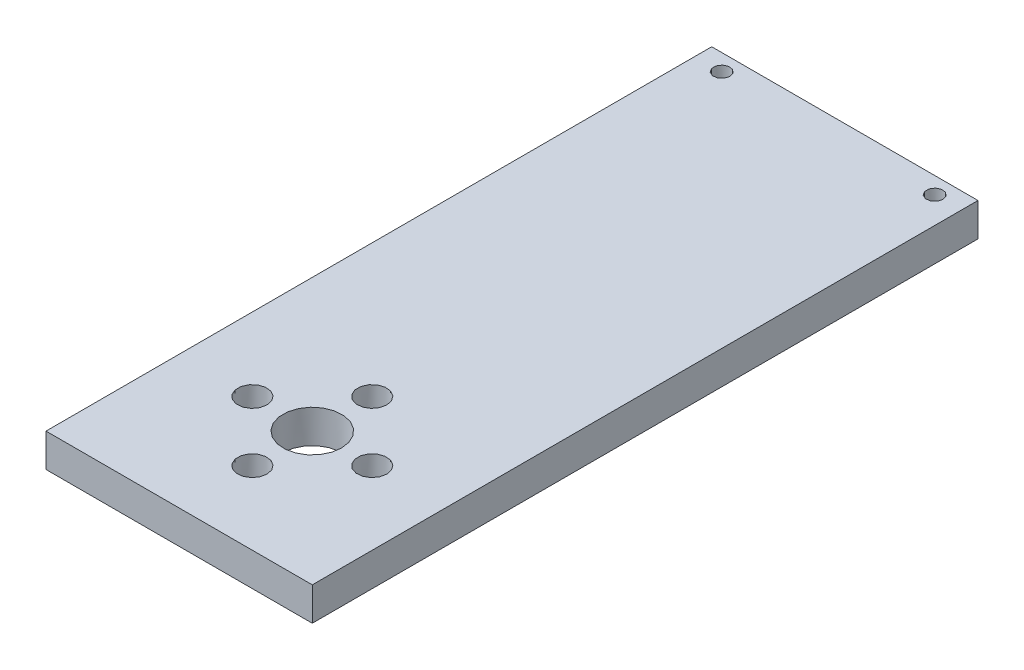
# Autodesk Inventor part: shoulder1_sidel_plate
Saved by Autodesk Inventor 2024 (Build 280153000, 153)
## iProperties
Created: 2025-08-06
Part Number: shoulder1_sidel_plate
Material: 一般
Document SubType Name: Modeling
Designer: HosodaLab2
Density: 1 g/cm^3
Appearance: 既定
Author: HosodaLab2
Autodesk Inventor part; units mm, degrees
ref_plane "YZ Plane" through (0, 0, 0) normal (1, 0, 0) x (0, 1, 0)
ref_plane "XZ Plane" through (0, 0, 0) normal (0, 1, 0) x (-1, 0, 0)
ref_plane "XY Plane" through (0, 0, 0) normal (0, 0, 1) x (1, 0, 0)
sketch "スケッチ1" plane through (0, 0, 0) normal (0, 1, 0) x (-1, 0, 0)
  line L0 (0, 0) -> (-40, 0)
  line L1 (-40, 0) -> (-40, -100)
  line L2 (-40, -100) -> (0, -100)
  line L3 (0, -100) -> (0, 0)
  dimension "d0" = 40
  dimension "d1" = 100
  constraints: 8 end point, 2 parallel, 1 horizontal, 1 perpendicular
  measures "d0" distance of L2.end L1.end
  measures "d1" distance of L1.end L0.end
extrude "押し出し1" add sketch "スケッチ1" along normal blind 5
sketch "スケッチ2" plane through (0, 5, 0) normal (0, 1, 0) x (1, 0, 0)
  line L0 (0, 0) -> (40, 0) construction
  line L1 (20, 0) -> (20, 100) construction
  line L2 (40, 100) -> (0, 100) construction
  point P0 (20, 20)
  dimension "d4" = 20
  constraints: 2 end point, 2 midpoint, 1 point on line
  measures "d4" distance from line of L0 point (20, 20)
hole "穴1" at (20, 5, -20) direction (0, -1, 0) diameter 8.8 end through all
sketch "スケッチ3" plane through (0, 5, 0) normal (0, 1, 0) x (1, 0, 0)
  circle A0 centre (20, 20) radius 4.4 construction
  circle A1 centre (20, 20) radius 9 construction
  point P0 (0, 0)
  point P1 (11, 20)
  point P2 (20, 11)
  point P3 (29, 20)
  point P4 (20, 29)
  dimension "d12" = 18
  dimension "d15" = 360
  constraints: 1 coincident, 1 horizontal alignment, 7 other
hole "穴2" at (11, 5, -20) at (20, 5, -11) at (29, 5, -20) at (20, 5, -29) direction (0, -1, 0) diameter 4.4 end through all
sketch "スケッチ4" plane through (0, 5, 0) normal (0, 1, 0) x (1, 0, 0)
  line L0 (40, 100) -> (0, 100) construction
  line L1 (0, 100) -> (40, 100) construction
  line L2 (40, 100) -> (40, 95) construction
  line L3 (40, 95) -> (0, 95) construction
  line L4 (0, 95) -> (0, 100) construction
  line L5 (0, 100) -> (0, 0) projected
  line L6 (0, 97.5) -> (40, 97.5) construction
  line L7 (40, 0) -> (40, 100) projected
  point P0 (4, 97.5)
  point P1 (36, 97.5)
  dimension "d25" = 5
  dimension "d26" = 4
  dimension "d27" = 4
  constraints: 10 end point, 3 point on line, 2 parallel, 1 horizontal, 1 midpoint, 1 perpendicular
  measures "d25" distance of L1.end L2.end
  measures "d26" distance from line of point (4, 97.5) L5
  measures "d27" distance from line of L7 point (36, 97.5)
hole "穴3" at (4, 5, -97.5) at (36, 5, -97.5) direction (0, -1, 0) diameter 2.459 end through all thread size "M3x0.5" class "6H" standard "ISO Metric profile"
